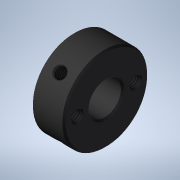
# Autodesk Inventor part: PSCTW10b
Saved by Autodesk Inventor 2021 (Build 250183000, 183)
## iProperties
Created: 2025-04-29
Part Number: PSCTW10b
Material: Generic
Catalog Web Link: www.cadenas.de
Description: SCTW, PSCTW, SSCTW-b-Shaft Collars - Set Screw, with 2 Holes
Vendor: MISUMI
Document SubType Name: Modeling
Designer: psAdmin
Manufacturer: MISUMI
Mass: 4.19026 g
Surface Area: 22.5732 cm^2
Volume: 4.19026 cm^3
Density: 1 g/cm^3
Appearance: PSOLRGB-175-175-175
Category: PARTsolutions
Company: MISUMI
Title: PSCTW10
Author: Cadenas PARTsolutions
Comments: Shaft Collars - Set Screw, with 2 Holes
PSOL_IDENT_0: {$CADENAS_DATA/23d-libs/misumi/metric/03_set_collars/sctw/sctw_b.prj},175 {VTYP=3D},{NB=PSCTW10b},{L
PSOL_IDENT_1: INA=PSCTW10},{NN=SCTW, PSCTW, SSCTW-b},{DATE=02.06.2021 03:00:04},{GEOMDATE=25.12.2015 07:47:56},{VE
PSOL_IDENT_2: RSION=},{LINEID=60},{WBVAR=MAT,ST},{WBNUMERIC=}  {NB=PSCTW10b},{LINA=PSCTW10},{KT=DUMMY},{PN=PSCTW10
PSOL_IDENT_3: },{TYPE=PSCTW},{MAT=1045},{ST=Electroless Nickel Plating},{AC=Set Screws 2 Pcs. (304 Stainless Steel
PSOL_IDENT_4: ) },{D=10},{B=10},{D1=26},{P=18},{M=M4x4},{THMD=4},{THDMIN=3.242},{M1=M4},{M1NDM=4},{C=0.5},{ST0='Bl
PSOL_IDENT_5: ack Oxide','Black Oxide','Electroless Nickel Plating','Electroless Nickel Plating'},{L=4}
NB: PSCTW10b
NN: SCTW, PSCTW, SSCTW-b
NT: Shaft Collars - Set Screw, with 2 Holes
NBSYN: $PN.b
LINA: PSCTW10
CATALOG: Misumi
PN: PSCTW10
MAT: S45C Equivalent
ST: Electroless Nickel Plating
AC: Set Screws 2 Pcs. (304 Stainless Steel)
D: 10
B: 10
D1: 26
P: 18
M: M4x4
M1: M4
SUPPLIER: MISUMI
ARTICLENO: PSCTW10b
BOMINFO: PSCTW10
CREATOR: CADENAS GmbH
Autodesk Inventor part; units mm, degrees
sketch "Sketch_1" plane through (0, 0, 0) normal (0, 0, 1) x (1, 0, 0)
  line L0 (0, 0) -> (-5, 0)
  line L1 (-5, 5.5) -> (-4.5, 5)
  line L2 (-4.5, 5) -> (4.5, 5)
  line L3 (4.5, 5) -> (5, 5.5)
  line L4 (5, 5.5) -> (5, 12.5)
  line L5 (5, 12.5) -> (4.5, 13)
  line L6 (4.5, 13) -> (-4.5, 13)
  line L7 (-4.5, 13) -> (-5, 12.5)
  line L8 (-5, 12.5) -> (-5, 5.5)
  constraints: 18 end point
revolve "Revolution1" add sketch "Sketch_1" angle 360 about axis through (0, 0, 0) along (1, 0, 0)
sketch "Sketch_2" plane through (0, 0, 0) normal (1, 0, 0) x (0, 1, 0)
  line L0 (10.1116, 10.1116) -> (2.6163, 2.6163)
  line L1 (2.6163, 2.6163) -> (1.2021, 4.0305)
  line L2 (1.2021, 4.0305) -> (2.1213, 4.9497)
  line L3 (2.1213, 4.9497) -> (2.6573, 4.9497)
  line L4 (2.6573, 4.9497) -> (7.7782, 10.0706)
  line L5 (7.7782, 10.0706) -> (7.7782, 10.6066)
  line L6 (7.7782, 10.6066) -> (8.6974, 11.5258)
  line L7 (8.6974, 11.5258) -> (10.1116, 10.1116)
  line L8 (10.1116, 10.1116) -> (2.6163, 2.6163)
  constraints: 18 end point
revolve "Revolution2" cut sketch "Sketch_2" angle 360 about axis through (0, 10.1116, 10.1116) along (0, 0.7071068, 0.7071068)
thread "Thread1" size "M4x0.7" class "6H" standard "ISO Metric profile" full length
sketch "Sketch_3" plane through (0, 0, 0) normal (1, 0, 0) x (0, 1, 0)
  line L0 (-10.1116, 10.1116) -> (-2.6163, 2.6163)
  line L1 (-2.6163, 2.6163) -> (-4.0305, 1.2021)
  line L2 (-4.0305, 1.2021) -> (-4.9497, 2.1213)
  line L3 (-4.9497, 2.1213) -> (-4.9497, 2.6573)
  line L4 (-4.9497, 2.6573) -> (-10.0706, 7.7782)
  line L5 (-10.0706, 7.7782) -> (-10.6066, 7.7782)
  line L6 (-10.6066, 7.7782) -> (-11.5258, 8.6974)
  line L7 (-11.5258, 8.6974) -> (-10.1116, 10.1116)
  line L8 (-10.1116, 10.1116) -> (-2.6163, 2.6163)
  constraints: 18 end point
revolve "Revolution3" cut sketch "Sketch_3" angle 360 about axis through (0, -10.1116, 10.1116) along (0, -0.7071068, 0.7071068)
thread "Thread2" size "M4x0.7" class "6H" standard "ISO Metric profile" full length
sketch "Sketch_5" plane through (0, 0, 0) normal (0, 1, 0) x (-1, 0, 0)
  line L0 (-5, -9) -> (5, -9)
  line L1 (5, -9) -> (5, -11)
  line L2 (5, -11) -> (4.621, -10.621)
  line L3 (4.621, -10.621) -> (-4.621, -10.621)
  line L4 (-4.621, -10.621) -> (-5, -11)
  line L5 (-5, -11) -> (-5, -9)
  line L6 (-5, -9) -> (5, -9)
  constraints: 14 end point
revolve "Revolution4" cut sketch "Sketch_5" angle 360 about axis through (5, 0, -9) along (1, 0, 0)
thread "Thread3" size "M4x0.7" class "6H" standard "ISO Metric profile" full length
sketch "Sketch_9" plane through (0, 0, 0) normal (0, 1, 0) x (-1, 0, 0)
  line L0 (-5, 9) -> (5, 9)
  line L1 (5, 9) -> (5, 7)
  line L2 (5, 7) -> (4.621, 7.379)
  line L3 (4.621, 7.379) -> (-4.621, 7.379)
  line L4 (-4.621, 7.379) -> (-5, 7)
  line L5 (-5, 7) -> (-5, 9)
  line L6 (-5, 9) -> (5, 9)
  constraints: 14 end point
revolve "Revolution5" cut sketch "Sketch_9" angle 360 about axis through (5, 0, 9) along (1, 0, 0)
thread "Thread4" size "M4x0.7" class "6H" standard "ISO Metric profile" full length
ref_plane "body_set_h_XY" through (0, -9.1924, 9.1924) normal (0, 0.7071068, -0.7071068) x (1, 0, 0)
ref_plane "body_set_h_YZ" through (0, -9.1924, 9.1924) normal (1, 0, 0) x (0, -0.7071068, -0.7071068)
ref_plane "body_set_h_ZX" through (0, -9.1924, 9.1924) normal (0, -0.7071068, -0.7071068) x (0, 0.7071068, -0.7071068)
ref_plane "body_set_v_XY" through (0, 9.1924, 9.1924) normal (0, 0.7071068, 0.7071068) x (1, 0, 0)
ref_plane "body_set_v_YZ" through (0, 9.1924, 9.1924) normal (1, 0, 0) x (0, 0.7071068, -0.7071068)
ref_plane "body_set_v_ZX" through (0, 9.1924, 9.1924) normal (0, 0.7071068, -0.7071068) x (0, 0.7071068, 0.7071068)
body "Solid1"
